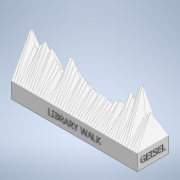
# Autodesk Inventor part: base_fourier
Saved by Autodesk Inventor 2020.1 (Build 241239000, 239)
## iProperties
Created: 2019-10-02
Part Number: base_fourier
Material: Generic
Document SubType Name: Modeling
Designer: Babynado
Density: 1 g/cm^3
Appearance: Default
Author: Babynado
Autodesk Inventor part; units mm, degrees
(part 1 of 3)
ref_plane "YZ Plane" through (0, 0, 0) normal (1, 0, 0) x (0, 1, 0)
ref_plane "XZ Plane" through (0, 0, 0) normal (0, 1, 0) x (-1, 0, 0)
ref_plane "XY Plane" through (0, 0, 0) normal (0, 0, 1) x (1, 0, 0)
sketch "Sketch1" plane through (0, 0, 0) normal (0, 1, 0) x (-1, 0, 0)
  line L0 (0, 50.8) -> (-203.2, 50.8) projected
  line L1 (0, 0) -> (0, 50.8) projected
  line L2 (-203.2, 0) -> (0, 0) projected
  line L3 (-203.2, 50.8) -> (-203.2, 0) projected
extrude "Extrusion1" add sketch "Sketch1" against normal blind 25.4
sketch "Sketch2" plane through (0, 0, 50.8) normal (0, 0, 1) x (1, 0, 0)
  line L0 (0, 0) -> (203.2, 0) projected
  line L1 (0, 0) -> (0, -25.4) projected
  line L2 (203.2, -25.4) -> (0, -25.4) projected
  line L3 (203.2, 0) -> (203.2, -25.4) projected
  line L4 (57.1858, -6.0743) -> (146.0142, -6.0743) construction
  line L5 (146.0142, -6.0743) -> (146.0142, -19.3257) construction
  line L6 (146.0142, -19.3257) -> (57.1858, -19.3257) construction
  line L7 (57.1858, -19.3257) -> (57.1858, -6.0743) construction
  line L8 (65.2204, -17.272) -> (59.9222, -17.272)
  line L9 (59.9222, -17.272) -> (59.9222, -8.128)
  line L10 (59.9222, -8.128) -> (61.1374, -8.128)
  line L11 (61.1374, -8.128) -> (61.1374, -16.1901)
  line L12 (61.1374, -16.1901) -> (65.2204, -16.1901)
  line L13 (65.2204, -16.1901) -> (65.2204, -17.272)
  line L14 (69.3626, -17.272) -> (65.8206, -17.272)
  line L15 (65.8206, -17.272) -> (65.8206, -16.3383)
  line L16 (65.8206, -16.3383) -> (66.984, -16.3383)
  line L17 (66.984, -16.3383) -> (66.984, -9.0617)
  line L18 (66.984, -9.0617) -> (65.8206, -9.0617)
  line L19 (65.8206, -9.0617) -> (65.8206, -8.128)
  line L20 (65.8206, -8.128) -> (69.3626, -8.128)
  line L21 (69.3626, -8.128) -> (69.3626, -9.0617)
  line L22 (69.3626, -9.0617) -> (68.1992, -9.0617)
  line L23 (68.1992, -9.0617) -> (68.1992, -16.3383)
  line L24 (68.1992, -16.3383) -> (69.3626, -16.3383)
  line L25 (69.3626, -16.3383) -> (69.3626, -17.272)
  spline S0 degree 2 poles (77.069, -14.4636) (77.069, -15.1453) (76.5503, -16.1901) (76.1205, -16.531) knots 0 0 0 1 2 2 2
  spline S1 degree 2 poles (76.1205, -16.531) (75.6018, -16.9311) (74.4236, -17.272) (73.49, -17.272) knots 0 0 0 1 2 2 2
  line L26 (73.49, -17.272) -> (70.8668, -17.272)
  line L27 (70.8668, -17.272) -> (70.8668, -8.128)
  line L28 (70.8668, -8.128) -> (73.2899, -8.128)
  spline S2 degree 2 poles (73.2899, -8.128) (74.268, -8.128) (75.2462, -8.254) (75.6908, -8.4985) knots 0 0 0 1 2 2 2
  spline S3 degree 2 poles (75.6908, -8.4985) (76.1872, -8.7579) (76.6392, -9.61) (76.6392, -10.188) knots 0 0 0 1 2 2 2
  spline S4 degree 2 poles (76.6392, -10.188) (76.6392, -10.8327) (75.9575, -11.8553) (75.3573, -12.1442) knots 0 0 0 1 2 2 2
  line L29 (75.3573, -12.1442) -> (75.3573, -12.1887)
  spline S5 degree 2 poles (75.3573, -12.1887) (76.1724, -12.411) (77.069, -13.5892) (77.069, -14.4636) knots 0 0 0 1 2 2 2
  spline S6 degree 2 poles (75.8019, -14.5155) (75.8019, -13.9968) (75.5055, -13.3299) (75.0609, -13.0927) knots 0 0 0 1 2 2 2
  spline S7 degree 2 poles (75.0609, -13.0927) (74.7719, -12.9445) (74.0902, -12.8556) (73.4603, -12.8556) knots 0 0 0 1 2 2 2
  line L30 (73.4603, -12.8556) -> (72.0821, -12.8556)
  line L31 (72.0821, -12.8556) -> (72.0821, -16.2346)
  line L32 (72.0821, -16.2346) -> (73.0676, -16.2346)
  spline S8 degree 2 poles (73.0676, -16.2346) (73.8679, -16.2346) (74.7867, -16.0864) (75.1424, -15.8493) knots 0 0 0 1 2 2 2
  spline S9 degree 2 poles (75.1424, -15.8493) (75.4833, -15.6047) (75.8019, -14.9971) (75.8019, -14.5155) knots 0 0 0 1 2 2 2
  spline S10 degree 2 poles (75.3721, -10.3584) (75.3721, -10.0324) (75.1498, -9.5433) (74.9053, -9.4025) knots 0 0 0 1 2 2 2
  spline S11 degree 2 poles (74.9053, -9.4025) (74.6089, -9.2395) (73.8901, -9.1654) (73.2454, -9.1654) knots 0 0 0 1 2 2 2
  line L33 (73.2454, -9.1654) -> (72.0821, -9.1654)
  line L34 (72.0821, -9.1654) -> (72.0821, -11.8404)
  line L35 (72.0821, -11.8404) -> (73.4603, -11.8404)
  spline S12 degree 2 poles (73.4603, -11.8404) (74.0309, -11.8404) (74.5718, -11.7219) (74.8608, -11.5366) knots 0 0 0 1 2 2 2
  spline S13 degree 2 poles (74.8608, -11.5366) (75.1424, -11.3588) (75.3721, -10.7882) (75.3721, -10.3584) knots 0 0 0 1 2 2 2
  line L36 (85.3535, -17.272) -> (83.7751, -17.272)
  line L37 (83.7751, -17.272) -> (80.8852, -13.6337)
  line L38 (80.8852, -13.6337) -> (79.4921, -13.6337)
  line L39 (79.4921, -13.6337) -> (79.4921, -17.272)
  line L40 (79.4921, -17.272) -> (78.2769, -17.272)
  line L41 (78.2769, -17.272) -> (78.2769, -8.128)
  line L42 (78.2769, -8.128) -> (80.6333, -8.128)
  spline S14 degree 2 poles (80.6333, -8.128) (81.4187, -8.128) (82.4784, -8.2984) (82.96, -8.6097) knots 0 0 0 1 2 2 2
  spline S15 degree 2 poles (82.96, -8.6097) (83.4417, -8.9209) (83.9974, -9.8916) (83.9974, -10.6104) knots 0 0 0 1 2 2 2
  spline S16 degree 2 poles (83.9974, -10.6104) (83.9974, -11.6107) (82.9748, -12.9668) (82.1005, -13.2928) knots 0 0 0 1 2 2 2
  line L43 (82.1005, -13.2928) -> (85.3535, -17.272)
  spline S17 degree 2 poles (82.7303, -10.7067) (82.7303, -10.3066) (82.4487, -9.6915) (82.1523, -9.4914) knots 0 0 0 1 2 2 2
  spline S18 degree 2 poles (82.1523, -9.4914) (81.893, -9.321) (81.2038, -9.1802) (80.7, -9.1802) knots 0 0 0 1 2 2 2
  line L44 (80.7, -9.1802) -> (79.4921, -9.1802)
  line L45 (79.4921, -9.1802) -> (79.4921, -12.6185)
  line L46 (79.4921, -12.6185) -> (80.5592, -12.6185)
  spline S19 degree 2 poles (80.5592, -12.6185) (81.0853, -12.6185) (81.9226, -12.4332) (82.2116, -12.1442) knots 0 0 0 1 2 2 2
  spline S20 degree 2 poles (82.2116, -12.1442) (82.4784, -11.8923) (82.7303, -11.1809) (82.7303, -10.7067) knots 0 0 0 1 2 2 2
  line L47 (85.0941, -17.272) -> (88.1767, -8.128)
  line L48 (88.1767, -8.128) -> (89.6735, -8.128)
  line L49 (89.6735, -8.128) -> (92.7561, -17.272)
  line L50 (92.7561, -17.272) -> (91.4742, -17.272)
  line L51 (91.4742, -17.272) -> (90.6442, -14.7155)
  line L52 (90.6442, -14.7155) -> (87.1541, -14.7155)
  line L53 (87.1541, -14.7155) -> (86.3242, -17.272)
  line L54 (86.3242, -17.272) -> (85.0941, -17.272)
  line L55 (90.3108, -13.6781) -> (88.8955, -9.3729)
  line L56 (88.8955, -9.3729) -> (87.4876, -13.6781)
  line L57 (87.4876, -13.6781) -> (90.3108, -13.6781)
  line L58 (100.6997, -17.272) -> (99.1213, -17.272)
  line L59 (99.1213, -17.272) -> (96.2314, -13.6337)
  line L60 (96.2314, -13.6337) -> (94.8383, -13.6337)
  line L61 (94.8383, -13.6337) -> (94.8383, -17.272)
  line L62 (94.8383, -17.272) -> (93.6231, -17.272)
  line L63 (93.6231, -17.272) -> (93.6231, -8.128)
  line L64 (93.6231, -8.128) -> (95.9795, -8.128)
  spline S21 degree 2 poles (95.9795, -8.128) (96.7649, -8.128) (97.8246, -8.2984) (98.3062, -8.6097) knots 0 0 0 1 2 2 2
  spline S22 degree 2 poles (98.3062, -8.6097) (98.7879, -8.9209) (99.3436, -9.8916) (99.3436, -10.6104) knots 0 0 0 1 2 2 2
  spline S23 degree 2 poles (99.3436, -10.6104) (99.3436, -11.6107) (98.3211, -12.9668) (97.4467, -13.2928) knots 0 0 0 1 2 2 2
  line L65 (97.4467, -13.2928) -> (100.6997, -17.272)
  spline S24 degree 2 poles (98.0765, -10.7067) (98.0765, -10.3066) (97.7949, -9.6915) (97.4985, -9.4914) knots 0 0 0 1 2 2 2
  spline S25 degree 2 poles (97.4985, -9.4914) (97.2392, -9.321) (96.55, -9.1802) (96.0462, -9.1802) knots 0 0 0 1 2 2 2
  line L66 (96.0462, -9.1802) -> (94.8383, -9.1802)
  line L67 (94.8383, -9.1802) -> (94.8383, -12.6185)
  line L68 (94.8383, -12.6185) -> (95.9054, -12.6185)
  spline S26 degree 2 poles (95.9054, -12.6185) (96.4315, -12.6185) (97.2688, -12.4332) (97.5578, -12.1442) knots 0 0 0 1 2 2 2
  spline S27 degree 2 poles (97.5578, -12.1442) (97.8246, -11.8923) (98.0765, -11.1809) (98.0765, -10.7067) knots 0 0 0 1 2 2 2
  line L69 (107.8281, -8.128) -> (104.7382, -13.2261)
  line L70 (104.7382, -13.2261) -> (104.7382, -17.272)
  line L71 (104.7382, -17.272) -> (103.5229, -17.272)
  line L72 (103.5229, -17.272) -> (103.5229, -13.3521)
  line L73 (103.5229, -13.3521) -> (100.4329, -8.128)
  line L74 (100.4329, -8.128) -> (101.7815, -8.128)
  line L75 (101.7815, -8.128) -> (104.1379, -12.1517)
  line L76 (104.1379, -12.1517) -> (106.5388, -8.128)
  line L77 (106.5388, -8.128) -> (107.8281, -8.128)
  line L78 (122.8483, -8.128) -> (120.5512, -17.272)
  line L79 (120.5512, -17.272) -> (119.1877, -17.272)
  line L80 (119.1877, -17.272) -> (117.3278, -9.6841)
  line L81 (117.3278, -9.6841) -> (115.5198, -17.272)
  line L82 (115.5198, -17.272) -> (114.1711, -17.272)
  line L83 (114.1711, -17.272) -> (111.837, -8.128)
  line L84 (111.837, -8.128) -> (113.0893, -8.128)
  line L85 (113.0893, -8.128) -> (114.927, -15.7085)
  line L86 (114.927, -15.7085) -> (116.7498, -8.128)
  line L87 (116.7498, -8.128) -> (117.9873, -8.128)
  line L88 (117.9873, -8.128) -> (119.825, -15.7974)
  line L89 (119.825, -15.7974) -> (121.6553, -8.128)
  line L90 (121.6553, -8.128) -> (122.8483, -8.128)
  line L91 (122.9521, -17.272) -> (126.0346, -8.128)
  line L92 (126.0346, -8.128) -> (127.5315, -8.128)
  line L93 (127.5315, -8.128) -> (130.614, -17.272)
  line L94 (130.614, -17.272) -> (129.3321, -17.272)
  line L95 (129.3321, -17.272) -> (128.5022, -14.7155)
  line L96 (128.5022, -14.7155) -> (125.012, -14.7155)
  line L97 (125.012, -14.7155) -> (124.1821, -17.272)
  line L98 (124.1821, -17.272) -> (122.9521, -17.272)
  line L99 (128.1687, -13.6781) -> (126.7534, -9.3729)
  line L100 (126.7534, -9.3729) -> (125.3455, -13.6781)
  line L101 (125.3455, -13.6781) -> (128.1687, -13.6781)
  line L102 (136.7792, -17.272) -> (131.481, -17.272)
  line L103 (131.481, -17.272) -> (131.481, -8.128)
  line L104 (131.481, -8.128) -> (132.6963, -8.128)
  line L105 (132.6963, -8.128) -> (132.6963, -16.1901)
  line L106 (132.6963, -16.1901) -> (136.7792, -16.1901)
  line L107 (136.7792, -16.1901) -> (136.7792, -17.272)
  line L108 (144.4041, -17.272) -> (142.8258, -17.272)
  line L109 (142.8258, -17.272) -> (139.4839, -13.0186)
  line L110 (139.4839, -13.0186) -> (138.9503, -13.6188)
  line L111 (138.9503, -13.6188) -> (138.9503, -17.272)
  line L112 (138.9503, -17.272) -> (137.7351, -17.272)
  line L113 (137.7351, -17.272) -> (137.7351, -8.128)
  line L114 (137.7351, -8.128) -> (138.9503, -8.128)
  line L115 (138.9503, -8.128) -> (138.9503, -12.3295)
  line L116 (138.9503, -12.3295) -> (142.6998, -8.128)
  line L117 (142.6998, -8.128) -> (144.1818, -8.128)
  line L118 (144.1818, -8.128) -> (140.3953, -12.2109)
  line L119 (140.3953, -12.2109) -> (144.4041, -17.272)
  dimension "d2" = 203.2
  dimension "d3" = 25.4
  dimension "d4" = 88.8284
  dimension "d5" = 13.2514
  dimension "d6" = 6.0743
  dimension "d7" = 57.1858
  constraints: 2 other
  measures "d2" distance of L0.start L0.end
  measures "d3" distance of L0.start L1.end
  measures "d4" distance of L4.start L4.end
  measures "d5" distance of L6.end L4.start
  measures "d6" distance between parallel lines of L0 L4
  measures "d7" distance between parallel lines of L1 L7
extrude "Extrusion2" cut sketch "Sketch2" against normal blind 5.08 contours L8 L9 L10 L11 L12 L13 | L14 L15 L16 L17 L18 L19 L20 L21 L22 L23 L24 L25 | S0 S1 L26 L27 L28 S2 S3 S4 L29 S5 | L36 L47 L43 | L43 L47 L48 L49 L50 L51 L52 L53 L54 | L36 L37 L38 L39 L40 L41 L42 S14 S15 S16 L43 L47 | L58 L59 L60 L61 L62 L63 L64 S21 S22 S23 L65 | L69 L70 L71 L72 L73 L74 L75 L76 L77 | L78 L79 L80 L81 L82 L83 L84 L85 L86 L87 L88 L89 L90 | L91 L92 L93 L94 L95 L96 L97 L98 | L102 L103 L104 L105 L106 L107 | L108 L109 L110 L111 L112 L113 L114 L115 L116 L117 L118 L119
sketch "Sketch3" plane through (0, -25.4, 0) normal (0, -1, 0) x (1, 0, 0)
  line L0 (203.2, 0) -> (203.2, 50.8) projected
  line L1 (203.2, 50.8) -> (0, 50.8) projected
  line L2 (0, 50.8) -> (0, 0) projected
  line L3 (0, 0) -> (203.2, 0) projected
  line L4 (6.672, 48.1679) -> (109.1926, 48.1679) construction
  line L5 (109.1926, 48.1679) -> (109.1926, 2.6321) construction
  line L6 (109.1926, 2.6321) -> (6.672, 2.6321) construction
  line L7 (6.672, 2.6321) -> (6.672, 48.1679) construction
  line L8 (115.8646, 37.7597) -> (196.528, 37.7597) construction
  line L9 (196.528, 37.7597) -> (196.528, 13.0403) construction
  line L10 (196.528, 13.0403) -> (115.8646, 13.0403) construction
  line L11 (115.8646, 13.0403) -> (115.8646, 37.7597) construction
  spline S0 degree 2 poles (22.1307, 39.4772) (22.1307, 38.2768) (20.6635, 36.9726) (19.426, 36.9726) knots 0 0 0 1 2 2 2
  spline S1 degree 2 poles (19.426, 36.9726) (19.1296, 36.9726) (18.144, 37.0764) (17.8106, 37.1505) knots 0 0 0 1 2 2 2
  line L12 (17.8106, 37.1505) -> (17.8106, 38.3213)
  line L13 (17.8106, 38.3213) -> (17.8773, 38.3213)
  spline S2 degree 2 poles (17.8773, 38.3213) (18.1292, 38.2323) (18.8776, 38.0249) (19.263, 38.0249) knots 0 0 0 1 2 2 2
  spline S3 degree 2 poles (19.263, 38.0249) (19.8261, 38.0249) (20.5004, 38.2842) (20.6561, 38.5213) knots 0 0 0 1 2 2 2
  spline S4 degree 2 poles (20.6561, 38.5213) (20.8265, 38.7659) (20.9154, 39.4772) (20.9154, 39.9441) knots 0 0 0 1 2 2 2
  line L14 (20.9154, 39.9441) -> (20.9154, 45.2719)
  line L15 (20.9154, 45.2719) -> (18.9814, 45.2719)
  line L16 (18.9814, 45.2719) -> (18.9814, 46.2426)
  line L17 (18.9814, 46.2426) -> (22.1307, 46.2426)
  line L18 (22.1307, 46.2426) -> (22.1307, 39.4772)
  spline S5 degree 2 poles (27.1176, 36.9059) (26.3099, 36.9059) (25.1095, 37.3283) (24.6871, 37.7507) knots 0 0 0 1 2 2 2
  spline S6 degree 2 poles (24.6871, 37.7507) (24.2055, 38.2249) (23.8127, 39.5587) (23.8127, 40.5369) knots 0 0 0 1 2 2 2
  line L19 (23.8127, 40.5369) -> (23.8127, 46.2426)
  line L20 (23.8127, 46.2426) -> (25.028, 46.2426)
  line L21 (25.028, 46.2426) -> (25.028, 40.5369)
  spline S7 degree 2 poles (25.028, 40.5369) (25.028, 39.8996) (25.191, 39.04) (25.4207, 38.6918) knots 0 0 0 1 2 2 2
  spline S8 degree 2 poles (25.4207, 38.6918) (25.6652, 38.3213) (26.51, 37.9433) (27.1176, 37.9433) knots 0 0 0 1 2 2 2
  spline S9 degree 2 poles (27.1176, 37.9433) (27.6882, 37.9433) (28.5774, 38.3213) (28.8219, 38.6918) knots 0 0 0 1 2 2 2
  spline S10 degree 2 poles (28.8219, 38.6918) (29.0516, 39.04) (29.2147, 39.8922) (29.2147, 40.5072) knots 0 0 0 1 2 2 2
  line L22 (29.2147, 40.5072) -> (29.2147, 46.2426)
  line L23 (29.2147, 46.2426) -> (30.4299, 46.2426)
  line L24 (30.4299, 46.2426) -> (30.4299, 40.5369)
  spline S11 degree 2 poles (30.4299, 40.5369) (30.4299, 39.581) (30.0446, 38.2175) (29.5555, 37.7507) knots 0 0 0 1 2 2 2
  spline S12 degree 2 poles (29.5555, 37.7507) (29.1183, 37.3209) (27.9624, 36.9059) (27.1176, 36.9059) knots 0 0 0 1 2 2 2
  spline S13 degree 2 poles (34.7203, 36.9356) (33.7274, 36.9356) (32.3343, 37.3505) (31.7193, 37.6469) knots 0 0 0 1 2 2 2
  line L25 (31.7193, 37.6469) -> (31.7193, 39.1734)
  line L26 (31.7193, 39.1734) -> (31.8082, 39.1734)
  spline S14 degree 2 poles (31.8082, 39.1734) (32.4084, 38.6103) (33.9274, 37.9878) (34.6314, 37.9878) knots 0 0 0 1 2 2 2
  spline S15 degree 2 poles (34.6314, 37.9878) (35.6392, 37.9878) (36.6692, 38.8251) (36.6692, 39.5143) knots 0 0 0 1 2 2 2
  spline S16 degree 2 poles (36.6692, 39.5143) (36.6692, 40.0626) (36.1282, 40.7443) (35.5428, 40.9148) knots 0 0 0 1 2 2 2
  spline S17 degree 2 poles (35.5428, 40.9148) (35.1205, 41.0333) (34.4165, 41.1964) (33.8904, 41.3297) knots 0 0 0 1 2 2 2
  spline S18 degree 2 poles (33.8904, 41.3297) (33.4162, 41.4557) (32.6677, 41.8336) (32.3787, 42.1374) knots 0 0 0 1 2 2 2
  spline S19 degree 2 poles (32.3787, 42.1374) (32.0972, 42.4412) (31.7859, 43.2564) (31.7859, 43.7899) knots 0 0 0 1 2 2 2
  spline S20 degree 2 poles (31.7859, 43.7899) (31.7859, 44.9014) (33.5199, 46.4056) (34.8611, 46.4056) knots 0 0 0 1 2 2 2
  spline S21 degree 2 poles (34.8611, 46.4056) (35.6318, 46.4056) (36.9952, 46.1018) (37.5806, 45.8128) knots 0 0 0 1 2 2 2
  line L27 (37.5806, 45.8128) -> (37.5806, 44.3605)
  line L28 (37.5806, 44.3605) -> (37.4917, 44.3605)
  spline S22 degree 2 poles (37.4917, 44.3605) (37.0545, 44.7606) (35.691, 45.3534) (34.9426, 45.3534) knots 0 0 0 1 2 2 2
  spline S23 degree 2 poles (34.9426, 45.3534) (34.0979, 45.3534) (33.0531, 44.5605) (33.0531, 43.9158) knots 0 0 0 1 2 2 2
  spline S24 degree 2 poles (33.0531, 43.9158) (33.0531, 43.3379) (33.6681, 42.6487) (34.2461, 42.4931) knots 0 0 0 1 2 2 2
  spline S25 degree 2 poles (34.2461, 42.4931) (34.6314, 42.3894) (35.7503, 42.1226) (36.1208, 42.0115) knots 0 0 0 1 2 2 2
  spline S26 degree 2 poles (36.1208, 42.0115) (37.0619, 41.7225) (37.9363, 40.5591) (37.9363, 39.7069) knots 0 0 0 1 2 2 2
  spline S27 degree 2 poles (37.9363, 39.7069) (37.9363, 39.166) (37.4991, 38.1286) (37.1064, 37.7655) knots 0 0 0 1 2 2 2
  spline S28 degree 2 poles (37.1064, 37.7655) (36.6692, 37.3654) (35.5577, 36.9356) (34.7203, 36.9356) knots 0 0 0 1 2 2 2
  line L29 (41.3079, 37.0986) -> (41.3079, 45.1607)
  line L30 (41.3079, 45.1607) -> (38.2401, 45.1607)
  line L31 (38.2401, 45.1607) -> (38.2401, 46.2426)
  line L32 (38.2401, 46.2426) -> (45.5909, 46.2426)
  line L33 (45.5909, 46.2426) -> (45.5909, 45.1607)
  line L34 (45.5909, 45.1607) -> (42.5231, 45.1607)
  line L35 (42.5231, 45.1607) -> (42.5231, 37.0986)
  line L36 (42.5231, 37.0986) -> (41.3079, 37.0986)
  line L37 (49.7034, 37.0986) -> (46.1614, 37.0986)
  line L38 (46.1614, 37.0986) -> (46.1614, 38.0323)
  line L39 (46.1614, 38.0323) -> (47.3248, 38.0323)
  line L40 (47.3248, 38.0323) -> (47.3248, 45.3089)
  line L41 (47.3248, 45.3089) -> (46.1614, 45.3089)
  line L42 (46.1614, 45.3089) -> (46.1614, 46.2426)
  line L43 (46.1614, 46.2426) -> (49.7034, 46.2426)
  line L44 (49.7034, 46.2426) -> (49.7034, 45.3089)
  line L45 (49.7034, 45.3089) -> (48.5401, 45.3089)
  line L46 (48.5401, 45.3089) -> (48.5401, 38.0323)
  line L47 (48.5401, 38.0323) -> (49.7034, 38.0323)
  line L48 (49.7034, 38.0323) -> (49.7034, 37.0986)
  line L49 (57.7508, 37.0986) -> (56.3873, 37.0986)
  line L50 (56.3873, 37.0986) -> (52.3414, 44.9829)
  line L51 (52.3414, 44.9829) -> (52.3414, 37.0986)
  line L52 (52.3414, 37.0986) -> (51.2077, 37.0986)
  line L53 (51.2077, 37.0986) -> (51.2077, 46.2426)
  line L54 (51.2077, 46.2426) -> (52.9342, 46.2426)
  line L55 (52.9342, 46.2426) -> (56.617, 39.003)
  line L56 (56.617, 39.003) -> (56.617, 46.2426)
  line L57 (56.617, 46.2426) -> (57.7508, 46.2426)
  line L58 (57.7508, 46.2426) -> (57.7508, 37.0986)
  line L59 (62.5451, 37.0986) -> (65.6276, 46.2426)
  line L60 (65.6276, 46.2426) -> (67.1245, 46.2426)
  line L61 (67.1245, 46.2426) -> (70.207, 37.0986)
  line L62 (70.207, 37.0986) -> (68.9251, 37.0986)
  line L63 (68.9251, 37.0986) -> (68.0952, 39.6551)
  line L64 (68.0952, 39.6551) -> (64.605, 39.6551)
  line L65 (64.605, 39.6551) -> (63.7751, 37.0986)
  line L66 (63.7751, 37.0986) -> (62.5451, 37.0986)
  line L67 (67.7617, 40.6925) -> (66.3464, 44.9977)
  line L68 (66.3464, 44.9977) -> (64.9385, 40.6925)
  line L69 (64.9385, 40.6925) -> (67.7617, 40.6925)
  line L70 (76.3722, 37.0986) -> (71.074, 37.0986)
  line L71 (71.074, 37.0986) -> (71.074, 46.2426)
  line L72 (71.074, 46.2426) -> (72.2893, 46.2426)
  line L73 (72.2893, 46.2426) -> (72.2893, 38.1805)
  line L74 (72.2893, 38.1805) -> (76.3722, 38.1805)
  line L75 (76.3722, 38.1805) -> (76.3722, 37.0986)
  line L76 (82.6263, 37.0986) -> (77.3281, 37.0986)
  line L77 (77.3281, 37.0986) -> (77.3281, 46.2426)
  line L78 (77.3281, 46.2426) -> (78.5433, 46.2426)
  line L79 (78.5433, 46.2426) -> (78.5433, 38.1805)
  line L80 (78.5433, 38.1805) -> (82.6263, 38.1805)
  line L81 (82.6263, 38.1805) -> (82.6263, 37.0986)
  line L82 (83.5822, 37.0986) -> (83.5822, 46.2426)
  line L83 (83.5822, 46.2426) -> (89.3027, 46.2426)
  line L84 (89.3027, 46.2426) -> (89.3027, 45.1607)
  line L85 (89.3027, 45.1607) -> (84.7974, 45.1607)
  line L86 (84.7974, 45.1607) -> (84.7974, 42.6561)
  line L87 (84.7974, 42.6561) -> (88.9989, 42.6561)
  line L88 (88.9989, 42.6561) -> (88.9989, 41.5743)
  line L89 (88.9989, 41.5743) -> (84.7974, 41.5743)
  line L90 (84.7974, 41.5743) -> (84.7974, 38.1805)
  line L91 (84.7974, 38.1805) -> (89.3027, 38.1805)
  line L92 (89.3027, 38.1805) -> (89.3027, 37.0986)
  line L93 (89.3027, 37.0986) -> (83.5822, 37.0986)
  line L94 (97.1796, 37.0986) -> (95.8162, 37.0986)
  line L95 (95.8162, 37.0986) -> (91.7703, 44.9829)
  line L96 (91.7703, 44.9829) -> (91.7703, 37.0986)
  line L97 (91.7703, 37.0986) -> (90.6365, 37.0986)
  line L98 (90.6365, 37.0986) -> (90.6365, 46.2426)
  line L99 (90.6365, 46.2426) -> (92.3631, 46.2426)
  line L100 (92.3631, 46.2426) -> (96.0459, 39.003)
  line L101 (96.0459, 39.003) -> (96.0459, 46.2426)
  line L102 (96.0459, 46.2426) -> (97.1796, 46.2426)
  line L103 (97.1796, 46.2426) -> (97.1796, 37.0986)
  line L104 (26.6545, 22.0432) -> (29.7371, 31.1872)
  line L105 (29.7371, 31.1872) -> (31.2339, 31.1872)
  line L106 (31.2339, 31.1872) -> (34.3165, 22.0432)
  line L107 (34.3165, 22.0432) -> (33.0345, 22.0432)
  line L108 (33.0345, 22.0432) -> (32.2046, 24.5997)
  line L109 (32.2046, 24.5997) -> (28.7145, 24.5997)
  line L110 (28.7145, 24.5997) -> (27.8846, 22.0432)
  line L111 (27.8846, 22.0432) -> (26.6545, 22.0432)
  line L112 (31.8712, 25.6371) -> (30.4558, 29.9424)
  line L113 (30.4558, 29.9424) -> (29.0479, 25.6371)
  line L114 (29.0479, 25.6371) -> (31.8712, 25.6371)
  line L115 (40.1037, 22.0432) -> (35.6429, 22.0432)
  line L116 (35.6429, 22.0432) -> (35.6429, 22.9769)
  line L117 (35.6429, 22.9769) -> (37.3027, 22.9769)
  line L118 (37.3027, 22.9769) -> (37.3027, 29.105)
  line L119 (37.3027, 29.105) -> (35.6429, 29.105)
  line L120 (35.6429, 29.105) -> (35.6429, 29.9424)
  spline S29 degree 2 poles (35.6429, 29.9424) (36.584, 29.9424) (37.4732, 30.4759) (37.5324, 31.2169) knots 0 0 0 1 2 2 2
  line L121 (37.5324, 31.2169) -> (38.4809, 31.2169)
  line L122 (38.4809, 31.2169) -> (38.4809, 22.9769)
  line L123 (38.4809, 22.9769) -> (40.1037, 22.9769)
  line L124 (40.1037, 22.9769) -> (40.1037, 22.0432)
  line L125 (47.6694, 25.1851) -> (46.5801, 25.1851)
  line L126 (46.5801, 25.1851) -> (46.5801, 22.0432)
  line L127 (46.5801, 22.0432) -> (45.4019, 22.0432)
  line L128 (45.4019, 22.0432) -> (45.4019, 25.1851)
  line L129 (45.4019, 25.1851) -> (41.3634, 25.1851)
  line L130 (41.3634, 25.1851) -> (41.3634, 26.4745)
  line L131 (41.3634, 26.4745) -> (45.4538, 31.1872)
  line L132 (45.4538, 31.1872) -> (46.5801, 31.1872)
  line L133 (46.5801, 31.1872) -> (46.5801, 26.1706)
  line L134 (46.5801, 26.1706) -> (47.6694, 26.1706)
  line L135 (47.6694, 26.1706) -> (47.6694, 25.1851)
  line L136 (45.4019, 26.1706) -> (45.4019, 29.7423)
  line L137 (45.4019, 29.7423) -> (42.3267, 26.1706)
  line L138 (42.3267, 26.1706) -> (45.4019, 26.1706)
  spline S30 degree 2 poles (54.1902, 24.948) (54.1902, 24.2885) (53.7679, 23.1622) (53.3825, 22.7472) knots 0 0 0 1 2 2 2
  spline S31 degree 2 poles (53.3825, 22.7472) (52.9972, 22.3322) (51.8487, 21.8506) (51.1373, 21.8506) knots 0 0 0 1 2 2 2
  spline S32 degree 2 poles (51.1373, 21.8506) (50.4852, 21.8506) (49.2107, 22.1396) (48.7438, 22.3693) knots 0 0 0 1 2 2 2
  line L139 (48.7438, 22.3693) -> (48.7438, 23.666)
  line L140 (48.7438, 23.666) -> (48.8328, 23.666)
  spline S33 degree 2 poles (48.8328, 23.666) (48.9736, 23.5623) (49.4997, 23.2955) (49.8183, 23.177) knots 0 0 0 1 2 2 2
  spline S34 degree 2 poles (49.8183, 23.177) (50.1814, 23.051) (50.7816, 22.9102) (51.1595, 22.9102) knots 0 0 0 1 2 2 2
  spline S35 degree 2 poles (51.1595, 22.9102) (51.53, 22.9102) (52.2266, 23.177) (52.4785, 23.466) knots 0 0 0 1 2 2 2
  spline S36 degree 2 poles (52.4785, 23.466) (52.7082, 23.7401) (52.9453, 24.4663) (52.9453, 24.9554) knots 0 0 0 1 2 2 2
  spline S37 degree 2 poles (52.9453, 24.9554) (52.9453, 25.4445) (52.6786, 26.0669) (52.4266, 26.2744) knots 0 0 0 1 2 2 2
  spline S38 degree 2 poles (52.4266, 26.2744) (52.1673, 26.5041) (51.3966, 26.6968) (50.9298, 26.6968) knots 0 0 0 1 2 2 2
  spline S39 degree 2 poles (50.9298, 26.6968) (50.4259, 26.6968) (49.4256, 26.5411) (49.1218, 26.4745) knots 0 0 0 1 2 2 2
  line L141 (49.1218, 26.4745) -> (49.1218, 31.1872)
  line L142 (49.1218, 31.1872) -> (54.1384, 31.1872)
  line L143 (54.1384, 31.1872) -> (54.1384, 30.1128)
  line L144 (54.1384, 30.1128) -> (50.3, 30.1128)
  line L145 (50.3, 30.1128) -> (50.3, 27.6749)
  spline S40 degree 2 poles (50.3, 27.6749) (50.5223, 27.7045) (50.952, 27.7268) (51.1299, 27.7268) knots 0 0 0 1 2 2 2
  spline S41 degree 2 poles (51.1299, 27.7268) (51.8338, 27.7268) (52.8045, 27.497) (53.2492, 27.1562) knots 0 0 0 1 2 2 2
  spline S42 degree 2 poles (53.2492, 27.1562) (53.7012, 26.8153) (54.1902, 25.7779) (54.1902, 24.948) knots 0 0 0 1 2 2 2
  spline S43 degree 2 poles (61.2891, 25.0073) (61.2891, 24.3033) (60.8222, 23.1103) (60.4295, 22.7102) knots 0 0 0 1 2 2 2
  spline S44 degree 2 poles (60.4295, 22.7102) (60.0219, 22.2878) (58.9993, 21.8506) (58.3843, 21.8506) knots 0 0 0 1 2 2 2
  spline S45 degree 2 poles (58.3843, 21.8506) (57.7693, 21.8506) (56.7541, 22.2655) (56.3688, 22.6805) knots 0 0 0 1 2 2 2
  spline S46 degree 2 poles (56.3688, 22.6805) (55.8945, 23.177) (55.361, 24.8442) (55.361, 26.0595) knots 0 0 0 1 2 2 2
  spline S47 degree 2 poles (55.361, 26.0595) (55.361, 27.2525) (55.8501, 29.1717) (56.3614, 29.8831) knots 0 0 0 1 2 2 2
  spline S48 degree 2 poles (56.3614, 29.8831) (56.8578, 30.5796) (58.4288, 31.3577) (59.4588, 31.3577) knots 0 0 0 1 2 2 2
  spline S49 degree 2 poles (59.4588, 31.3577) (59.7626, 31.3577) (60.2961, 31.2984) (60.4962, 31.2317) knots 0 0 0 1 2 2 2
  line L146 (60.4962, 31.2317) -> (60.4962, 30.0535)
  line L147 (60.4962, 30.0535) -> (60.4443, 30.0535)
  spline S50 degree 2 poles (60.4443, 30.0535) (60.2739, 30.1424) (59.6514, 30.298) (59.2957, 30.298) knots 0 0 0 1 2 2 2
  spline S51 degree 2 poles (59.2957, 30.298) (58.1546, 30.298) (56.7541, 28.7568) (56.6207, 27.2451) knots 0 0 0 1 2 2 2
  spline S52 degree 2 poles (56.6207, 27.2451) (57.0579, 27.5489) (57.9768, 27.8824) (58.5251, 27.8824) knots 0 0 0 1 2 2 2
  spline S53 degree 2 poles (58.5251, 27.8824) (59.0586, 27.8824) (59.8589, 27.6675) (60.2961, 27.3414) knots 0 0 0 1 2 2 2
  spline S54 degree 2 poles (60.2961, 27.3414) (60.8, 26.9635) (61.2891, 25.7927) (61.2891, 25.0073) knots 0 0 0 1 2 2 2
  spline S55 degree 2 poles (60.0442, 24.9554) (60.0442, 25.5186) (59.7478, 26.2818) (59.4217, 26.5486) knots 0 0 0 1 2 2 2
  spline S56 degree 2 poles (59.4217, 26.5486) (59.1772, 26.7412) (58.5696, 26.8672) (58.2509, 26.8672) knots 0 0 0 1 2 2 2
  spline S57 degree 2 poles (58.2509, 26.8672) (57.8212, 26.8672) (57.0135, 26.6078) (56.6207, 26.3633) knots 0 0 0 1 2 2 2
  spline S58 degree 2 poles (56.6207, 26.3633) (56.6133, 26.2299) (56.5985, 25.978) (56.5985, 25.7853) knots 0 0 0 1 2 2 2
  spline S59 degree 2 poles (56.5985, 25.7853) (56.5985, 24.8368) (56.969, 23.6735) (57.2506, 23.3696) knots 0 0 0 1 2 2 2
  spline S60 degree 2 poles (57.2506, 23.3696) (57.5099, 23.0807) (58.0731, 22.8509) (58.3917, 22.8509) knots 0 0 0 1 2 2 2
  spline S61 degree 2 poles (58.3917, 22.8509) (59.1327, 22.8509) (60.0442, 23.9032) (60.0442, 24.9554) knots 0 0 0 1 2 2 2
  spline S62 degree 2 poles (68.1508, 25.0073) (68.1508, 24.3033) (67.6839, 23.1103) (67.2912, 22.7102) knots 0 0 0 1 2 2 2
  spline S63 degree 2 poles (67.2912, 22.7102) (66.8836, 22.2878) (65.8611, 21.8506) (65.246, 21.8506) knots 0 0 0 1 2 2 2
  spline S64 degree 2 poles (65.246, 21.8506) (64.631, 21.8506) (63.6158, 22.2655) (63.2305, 22.6805) knots 0 0 0 1 2 2 2
  spline S65 degree 2 poles (63.2305, 22.6805) (62.7562, 23.177) (62.2227, 24.8442) (62.2227, 26.0595) knots 0 0 0 1 2 2 2
  spline S66 degree 2 poles (62.2227, 26.0595) (62.2227, 27.2525) (62.7118, 29.1717) (63.2231, 29.8831) knots 0 0 0 1 2 2 2
  spline S67 degree 2 poles (63.2231, 29.8831) (63.7195, 30.5796) (65.2905, 31.3577) (66.3205, 31.3577) knots 0 0 0 1 2 2 2
  spline S68 degree 2 poles (66.3205, 31.3577) (66.6243, 31.3577) (67.1578, 31.2984) (67.3579, 31.2317) knots 0 0 0 1 2 2 2
  line L148 (67.3579, 31.2317) -> (67.3579, 30.0535)
  line L149 (67.3579, 30.0535) -> (67.306, 30.0535)
  spline S69 degree 2 poles (67.306, 30.0535) (67.1356, 30.1424) (66.5131, 30.298) (66.1575, 30.298) knots 0 0 0 1 2 2 2
  spline S70 degree 2 poles (66.1575, 30.298) (65.0163, 30.298) (63.6158, 28.7568) (63.4824, 27.2451) knots 0 0 0 1 2 2 2
  spline S71 degree 2 poles (63.4824, 27.2451) (63.9196, 27.5489) (64.8385, 27.8824) (65.3868, 27.8824) knots 0 0 0 1 2 2 2
  spline S72 degree 2 poles (65.3868, 27.8824) (65.9203, 27.8824) (66.7206, 27.6675) (67.1578, 27.3414) knots 0 0 0 1 2 2 2
  spline S73 degree 2 poles (67.1578, 27.3414) (67.6617, 26.9635) (68.1508, 25.7927) (68.1508, 25.0073) knots 0 0 0 1 2 2 2
  spline S74 degree 2 poles (66.9059, 24.9554) (66.9059, 25.5186) (66.6095, 26.2818) (66.2834, 26.5486) knots 0 0 0 1 2 2 2
  spline S75 degree 2 poles (66.2834, 26.5486) (66.0389, 26.7412) (65.4313, 26.8672) (65.1126, 26.8672) knots 0 0 0 1 2 2 2
  spline S76 degree 2 poles (65.1126, 26.8672) (64.6829, 26.8672) (63.8752, 26.6078) (63.4824, 26.3633) knots 0 0 0 1 2 2 2
  spline S77 degree 2 poles (63.4824, 26.3633) (63.475, 26.2299) (63.4602, 25.978) (63.4602, 25.7853) knots 0 0 0 1 2 2 2
  spline S78 degree 2 poles (63.4602, 25.7853) (63.4602, 24.8368) (63.8307, 23.6735) (64.1123, 23.3696) knots 0 0 0 1 2 2 2
  spline S79 degree 2 poles (64.1123, 23.3696) (64.3716, 23.0807) (64.9348, 22.8509) (65.2534, 22.8509) knots 0 0 0 1 2 2 2
  spline S80 degree 2 poles (65.2534, 22.8509) (65.9944, 22.8509) (66.9059, 23.9032) (66.9059, 24.9554) knots 0 0 0 1 2 2 2
  spline S81 degree 2 poles (74.9235, 26.6152) (74.9235, 24.1551) (73.4934, 21.8506) (72.004, 21.8506) knots 0 0 0 1 2 2 2
  spline S82 degree 2 poles (72.004, 21.8506) (70.4923, 21.8506) (69.077, 24.1996) (69.077, 26.6078) knots 0 0 0 1 2 2 2
  spline S83 degree 2 poles (69.077, 26.6078) (69.077, 29.0828) (70.5072, 31.3725) (72.004, 31.3725) knots 0 0 0 1 2 2 2
  spline S84 degree 2 poles (72.004, 31.3725) (73.5082, 31.3725) (74.9235, 29.0013) (74.9235, 26.6152) knots 0 0 0 1 2 2 2
  spline S85 degree 2 poles (73.3526, 23.8291) (73.5305, 24.2811) (73.6787, 25.6742) (73.6787, 26.6152) knots 0 0 0 1 2 2 2
  spline S86 degree 2 poles (73.6787, 26.6152) (73.6787, 27.5563) (73.5305, 28.942) (73.3452, 29.4088) knots 0 0 0 1 2 2 2
  spline S87 degree 2 poles (73.3452, 29.4088) (73.16, 29.8757) (72.5153, 30.3573) (72.004, 30.3573) knots 0 0 0 1 2 2 2
  spline S88 degree 2 poles (72.004, 30.3573) (71.4927, 30.3573) (70.8332, 29.8757) (70.6405, 29.394) knots 0 0 0 1 2 2 2
  spline S89 degree 2 poles (70.6405, 29.394) (70.4553, 28.9272) (70.3219, 27.5045) (70.3219, 26.6078) knots 0 0 0 1 2 2 2
  spline S90 degree 2 poles (70.3219, 26.6078) (70.3219, 25.6445) (70.4405, 24.3552) (70.6331, 23.8513) knots 0 0 0 1 2 2 2
  spline S91 degree 2 poles (70.6331, 23.8513) (70.811, 23.3771) (71.4705, 22.8658) (72.004, 22.8658) knots 0 0 0 1 2 2 2
  spline S92 degree 2 poles (72.004, 22.8658) (72.5079, 22.8658) (73.1674, 23.3474) (73.3526, 23.8291) knots 0 0 0 1 2 2 2
  line L150 (81.8371, 29.8164) -> (77.8802, 22.0432)
  line L151 (77.8802, 22.0432) -> (76.576, 22.0432)
  line L152 (76.576, 22.0432) -> (80.7553, 30.1128)
  line L153 (80.7553, 30.1128) -> (76.035, 30.1128)
  line L154 (76.035, 30.1128) -> (76.035, 31.1872)
  line L155 (76.035, 31.1872) -> (81.8371, 31.1872)
  line L156 (81.8371, 31.1872) -> (81.8371, 29.8164)
  line L157 (88.1357, 22.0432) -> (83.6748, 22.0432)
  line L158 (83.6748, 22.0432) -> (83.6748, 22.9769)
  line L159 (83.6748, 22.9769) -> (85.3347, 22.9769)
  line L160 (85.3347, 22.9769) -> (85.3347, 29.105)
  line L161 (85.3347, 29.105) -> (83.6748, 29.105)
  line L162 (83.6748, 29.105) -> (83.6748, 29.9424)
  spline S93 degree 2 poles (83.6748, 29.9424) (84.6159, 29.9424) (85.5051, 30.4759) (85.5644, 31.2169) knots 0 0 0 1 2 2 2
  line L163 (85.5644, 31.2169) -> (86.5129, 31.2169)
  line L164 (86.5129, 31.2169) -> (86.5129, 22.9769)
  line L165 (86.5129, 22.9769) -> (88.1357, 22.9769)
  line L166 (88.1357, 22.9769) -> (88.1357, 22.0432)
  spline S94 degree 2 poles (11.8048, 6.7952) (11.8048, 5.6244) (10.545, 4.3944) (9.4409, 4.3944) knots 0 0 0 1 2 2 2
  spline S95 degree 2 poles (9.4409, 4.3944) (9.2483, 4.3944) (8.774, 4.4314) (8.5443, 4.4685) knots 0 0 0 1 2 2 2
  line L167 (8.5443, 4.4685) -> (8.5443, 5.5059)
  line L168 (8.5443, 5.5059) -> (8.611, 5.5059)
  spline S96 degree 2 poles (8.611, 5.5059) (8.7444, 5.4762) (9.0704, 5.417) (9.2186, 5.417) knots 0 0 0 1 2 2 2
  spline S97 degree 2 poles (9.2186, 5.417) (9.6781, 5.417) (10.2783, 5.6467) (10.4191, 5.8912) knots 0 0 0 1 2 2 2
  spline S98 degree 2 poles (10.4191, 5.8912) (10.5599, 6.1135) (10.6488, 6.7878) (10.6488, 7.2695) knots 0 0 0 1 2 2 2
  line L169 (10.6488, 7.2695) -> (10.6488, 12.8937)
  line L170 (10.6488, 12.8937) -> (9.4113, 12.8937)
  line L171 (9.4113, 12.8937) -> (9.4113, 13.8496)
  line L172 (9.4113, 13.8496) -> (11.8048, 13.8496)
  line L173 (11.8048, 13.8496) -> (11.8048, 6.7952)
  line L174 (11.8122, 14.9907) -> (10.5006, 14.9907)
  line L175 (10.5006, 14.9907) -> (10.5006, 16.1912)
  line L176 (10.5006, 16.1912) -> (11.8122, 16.1912)
  line L177 (11.8122, 16.1912) -> (11.8122, 14.9907)
  spline S99 degree 2 poles (19.2296, 10.5299) (19.2296, 8.8478) (17.5994, 6.7952) (16.3693, 6.7952) knots 0 0 0 1 2 2 2
  spline S100 degree 2 poles (16.3693, 6.7952) (15.8136, 6.7952) (15.0207, 7.0694) (14.6354, 7.3065) knots 0 0 0 1 2 2 2
  line L178 (14.6354, 7.3065) -> (14.5613, 6.9879)
  line L179 (14.5613, 6.9879) -> (13.4794, 6.9879)
  line L180 (13.4794, 6.9879) -> (13.4794, 16.5394)
  line L181 (13.4794, 16.5394) -> (14.6354, 16.5394)
  line L182 (14.6354, 16.5394) -> (14.6354, 13.1308)
  spline S101 degree 2 poles (14.6354, 13.1308) (15.0726, 13.5236) (16.0878, 14.0423) (16.7324, 14.0423) knots 0 0 0 1 2 2 2
  spline S102 degree 2 poles (16.7324, 14.0423) (17.8958, 14.0423) (19.2296, 12.1823) (19.2296, 10.5299) knots 0 0 0 1 2 2 2
  spline S103 degree 2 poles (18.0366, 10.441) (18.0366, 11.671) (17.2882, 12.9456) (16.4583, 12.9456) knots 0 0 0 1 2 2 2
  spline S104 degree 2 poles (16.4583, 12.9456) (15.9914, 12.9456) (15.0281, 12.501) (14.6354, 12.1601) knots 0 0 0 1 2 2 2
  line L183 (14.6354, 12.1601) -> (14.6354, 8.2254)
  spline S105 degree 2 poles (14.6354, 8.2254) (15.0726, 8.0105) (15.7469, 7.8326) (16.147, 7.8326) knots 0 0 0 1 2 2 2
  spline S106 degree 2 poles (16.147, 7.8326) (17.0288, 7.8326) (18.0366, 9.0849) (18.0366, 10.441) knots 0 0 0 1 2 2 2
  spline S107 degree 2 poles (24.2536, 7.7141) (24.1128, 7.6103) (23.6386, 7.2398) (23.4163, 7.1287) knots 0 0 0 1 2 2 2
  spline S108 degree 2 poles (23.4163, 7.1287) (23.1125, 6.9657) (22.5419, 6.7952) (22.0232, 6.7952) knots 0 0 0 1 2 2 2
  spline S109 degree 2 poles (22.0232, 6.7952) (21.6008, 6.7952) (20.8376, 7.1139) (20.5486, 7.4029) knots 0 0 0 1 2 2 2
  spline S110 degree 2 poles (20.5486, 7.4029) (20.2744, 7.6844) (19.941, 8.5144) (19.941, 8.9738) knots 0 0 0 1 2 2 2
  spline S111 degree 2 poles (19.941, 8.9738) (19.941, 9.6852) (20.5412, 10.6929) (21.1933, 10.9819) knots 0 0 0 1 2 2 2
  spline S112 degree 2 poles (21.1933, 10.9819) (21.7713, 11.2487) (23.3422, 11.4487) (24.2536, 11.5006) knots 0 0 0 1 2 2 2
  line L184 (24.2536, 11.5006) -> (24.2536, 11.7229)
  spline S113 degree 2 poles (24.2536, 11.7229) (24.2536, 12.1231) (24.0091, 12.6195) (23.7868, 12.7603) knots 0 0 0 1 2 2 2
  spline S114 degree 2 poles (23.7868, 12.7603) (23.5645, 12.9011) (22.9272, 12.99) (22.5864, 12.99) knots 0 0 0 1 2 2 2
  spline S115 degree 2 poles (22.5864, 12.99) (22.1862, 12.99) (21.1044, 12.7529) (20.5634, 12.5232) knots 0 0 0 1 2 2 2
  line L185 (20.5634, 12.5232) -> (20.4967, 12.5232)
  line L186 (20.4967, 12.5232) -> (20.4967, 13.7014)
  spline S116 degree 2 poles (20.4967, 13.7014) (20.8154, 13.7903) (22.0084, 14.0126) (22.5938, 14.0126) knots 0 0 0 1 2 2 2
  spline S117 degree 2 poles (22.5938, 14.0126) (23.3051, 14.0126) (24.2759, 13.7903) (24.6612, 13.5013) knots 0 0 0 1 2 2 2
  spline S118 degree 2 poles (24.6612, 13.5013) (25.0391, 13.2197) (25.4096, 12.3231) (25.4096, 11.6785) knots 0 0 0 1 2 2 2
  line L187 (25.4096, 11.6785) -> (25.4096, 6.9879)
  line L188 (25.4096, 6.9879) -> (24.2536, 6.9879)
  line L189 (24.2536, 6.9879) -> (24.2536, 7.7141)
  line L190 (24.2536, 8.6774) -> (24.2536, 10.5818)
  spline S119 degree 2 poles (24.2536, 10.5818) (23.8387, 10.5447) (22.5864, 10.4187) (22.1936, 10.3002) knots 0 0 0 1 2 2 2
  spline S120 degree 2 poles (22.1936, 10.3002) (21.7342, 10.1594) (21.134, 9.574) (21.134, 9.0553) knots 0 0 0 1 2 2 2
  spline S121 degree 2 poles (21.134, 9.0553) (21.134, 8.4625) (21.8009, 7.8623) (22.4382, 7.8623) knots 0 0 0 1 2 2 2
  spline S122 degree 2 poles (22.4382, 7.8623) (22.9791, 7.8623) (23.8683, 8.3291) (24.2536, 8.6774) knots 0 0 0 1 2 2 2
  line L191 (28.2106, 6.9879) -> (27.0546, 6.9879)
  line L192 (27.0546, 6.9879) -> (27.0546, 16.5394)
  line L193 (27.0546, 16.5394) -> (28.2106, 16.5394)
  line L194 (28.2106, 16.5394) -> (28.2106, 6.9879)
  line L195 (31.0857, 6.9879) -> (29.9297, 6.9879)
  line L196 (29.9297, 6.9879) -> (29.9297, 16.5394)
  line L197 (29.9297, 16.5394) -> (31.0857, 16.5394)
  line L198 (31.0857, 16.5394) -> (31.0857, 6.9879)
  spline S123 degree 2 poles (35.7614, 6.8323) (34.1164, 6.8323) (32.3084, 8.6774) (32.3084, 10.3817) knots 0 0 0 1 2 2 2
  spline S124 degree 2 poles (32.3084, 10.3817) (32.3084, 12.0564) (34.0645, 14.0423) (35.4799, 14.0423) knots 0 0 0 1 2 2 2
  spline S125 degree 2 poles (35.4799, 14.0423) (36.1171, 14.0423) (37.1027, 13.6718) (37.4657, 13.279) knots 0 0 0 1 2 2 2
  spline S126 degree 2 poles (37.4657, 13.279) (37.8363, 12.8863) (38.229, 11.7526) (38.229, 10.93) knots 0 0 0 1 2 2 2
  line L199 (38.229, 10.93) -> (38.229, 10.3002)
  line L200 (38.229, 10.3002) -> (33.4791, 10.3002)
  spline S127 degree 2 poles (33.4791, 10.3002) (33.4791, 9.1072) (34.6796, 7.84) (35.7466, 7.84) knots 0 0 0 1 2 2 2
  spline S128 degree 2 poles (35.7466, 7.84) (36.1245, 7.84) (36.8581, 8.0105) (37.1545, 8.1439) knots 0 0 0 1 2 2 2
  spline S129 degree 2 poles (37.1545, 8.1439) (37.4657, 8.2921) (37.8955, 8.5514) (38.0363, 8.67) knots 0 0 0 1 2 2 2
  line L201 (38.0363, 8.67) -> (38.103, 8.67)
  line L202 (38.103, 8.67) -> (38.103, 7.4103)
  spline S130 degree 2 poles (38.103, 7.4103) (37.9029, 7.3288) (37.2953, 7.0916) (37.0582, 7.0249) knots 0 0 0 1 2 2 2
  spline S131 degree 2 poles (37.0582, 7.0249) (36.7247, 6.9286) (36.1764, 6.8323) (35.7614, 6.8323) knots 0 0 0 1 2 2 2
  spline S132 degree 2 poles (37.1027, 11.182) (37.0878, 11.6488) (36.8952, 12.3305) (36.7099, 12.5602) knots 0 0 0 1 2 2 2
  spline S133 degree 2 poles (36.7099, 12.5602) (36.5099, 12.8196) (35.88, 13.0938) (35.4132, 13.0938) knots 0 0 0 1 2 2 2
  spline S134 degree 2 poles (35.4132, 13.0938) (34.9537, 13.0938) (34.3091, 12.8196) (34.0423, 12.5528) knots 0 0 0 1 2 2 2
  spline S135 degree 2 poles (34.0423, 12.5528) (33.783, 12.2787) (33.5162, 11.6192) (33.4791, 11.182) knots 0 0 0 1 2 2 2
  line L203 (33.4791, 11.182) -> (37.1027, 11.182)
  line L204 (44.7869, 6.9879) -> (43.6309, 6.9879)
  line L205 (43.6309, 6.9879) -> (43.6309, 10.9004)
  spline S136 degree 2 poles (43.6309, 10.9004) (43.6309, 11.3746) (43.542, 12.1897) (43.4086, 12.4343) knots 0 0 0 1 2 2 2
  spline S137 degree 2 poles (43.4086, 12.4343) (43.2678, 12.6936) (42.7639, 12.9456) (42.3342, 12.9456) knots 0 0 0 1 2 2 2
  spline S138 degree 2 poles (42.3342, 12.9456) (41.9044, 12.9456) (40.9929, 12.4861) (40.5557, 12.1156) knots 0 0 0 1 2 2 2
  line L206 (40.5557, 12.1156) -> (40.5557, 6.9879)
  line L207 (40.5557, 6.9879) -> (39.3998, 6.9879)
  line L208 (39.3998, 6.9879) -> (39.3998, 13.8496)
  line L209 (39.3998, 13.8496) -> (40.5557, 13.8496)
  line L210 (40.5557, 13.8496) -> (40.5557, 13.0864)
  spline S139 degree 2 poles (40.5557, 13.0864) (41.0744, 13.5532) (42.0748, 14.0423) (42.638, 14.0423) knots 0 0 0 1 2 2 2
  spline S140 degree 2 poles (42.638, 14.0423) (43.6457, 14.0423) (44.7869, 12.7085) (44.7869, 11.4413) knots 0 0 0 1 2 2 2
  line L211 (44.7869, 11.4413) -> (44.7869, 6.9879)
  spline S141 degree 2 poles (56.2502, 11.0634) (56.2502, 10.2113) (55.7834, 8.6181) (55.3462, 7.9586) knots 0 0 0 1 2 2 2
  line L212 (55.3462, 7.9586) -> (52.7675, 7.9586)
  line L213 (52.7675, 7.9586) -> (52.6119, 8.67)
  spline S142 degree 2 poles (52.6119, 8.67) (52.1969, 8.3217) (51.5078, 7.9067) (50.9076, 7.9067) knots 0 0 0 1 2 2 2
  spline S143 degree 2 poles (50.9076, 7.9067) (49.9665, 7.9067) (48.7587, 9.4258) (48.7587, 10.8633) knots 0 0 0 1 2 2 2
  spline S144 degree 2 poles (48.7587, 10.8633) (48.7587, 12.3083) (50.2407, 13.9163) (51.1966, 13.9163) knots 0 0 0 1 2 2 2
  spline S145 degree 2 poles (51.1966, 13.9163) (51.6412, 13.9163) (52.2784, 13.694) (52.6045, 13.5087) knots 0 0 0 1 2 2 2
  line L214 (52.6045, 13.5087) -> (52.6045, 13.8051)
  line L215 (52.6045, 13.8051) -> (53.5752, 13.8051)
  line L216 (53.5752, 13.8051) -> (53.5752, 8.6403)
  line L217 (53.5752, 8.6403) -> (54.9683, 8.6403)
  spline S146 degree 2 poles (54.9683, 8.6403) (55.2054, 9.0775) (55.4055, 10.4632) (55.4055, 11.0264) knots 0 0 0 1 2 2 2
  spline S147 degree 2 poles (55.4055, 11.0264) (55.4055, 13.0345) (53.3603, 15.4798) (51.4411, 15.4798) knots 0 0 0 1 2 2 2
  spline S148 degree 2 poles (51.4411, 15.4798) (49.6256, 15.4798) (47.2618, 12.8344) (47.2618, 10.9449) knots 0 0 0 1 2 2 2
  spline S149 degree 2 poles (47.2618, 10.9449) (47.2618, 8.9219) (49.5589, 6.4099) (51.4115, 6.4099) knots 0 0 0 1 2 2 2
  spline S150 degree 2 poles (51.4115, 6.4099) (51.9079, 6.4099) (53.012, 6.5433) (53.5011, 6.6915) knots 0 0 0 1 2 2 2
  line L218 (53.5011, 6.6915) -> (53.5011, 5.8245)
  spline S151 degree 2 poles (53.5011, 5.8245) (52.9824, 5.6985) (51.9228, 5.6022) (51.4041, 5.6022) knots 0 0 0 1 2 2 2
  spline S152 degree 2 poles (51.4041, 5.6022) (49.2329, 5.6022) (46.38, 8.5885) (46.38, 10.9597) knots 0 0 0 1 2 2 2
  spline S153 degree 2 poles (46.38, 10.9597) (46.38, 13.2123) (49.3218, 16.3097) (51.4337, 16.3097) knots 0 0 0 1 2 2 2
  spline S154 degree 2 poles (51.4337, 16.3097) (53.6938, 16.3097) (56.2502, 13.3976) (56.2502, 11.0634) knots 0 0 0 1 2 2 2
  line L219 (52.5897, 9.4925) -> (52.5897, 12.6714)
  spline S155 degree 2 poles (52.5897, 12.6714) (52.2488, 12.8492) (51.6708, 13.0049) (51.3522, 13.0049) knots 0 0 0 1 2 2 2
  spline S156 degree 2 poles (51.3522, 13.0049) (50.6556, 13.0049) (49.8109, 11.9674) (49.8109, 10.8782) knots 0 0 0 1 2 2 2
  spline S157 degree 2 poles (49.8109, 10.8782) (49.8109, 9.9) (50.4482, 8.8552) (51.1521, 8.8552) knots 0 0 0 1 2 2 2
  spline S158 degree 2 poles (51.1521, 8.8552) (51.5226, 8.8552) (52.2562, 9.2109) (52.5897, 9.4925) knots 0 0 0 1 2 2 2
  line L220 (63.1786, 6.9879) -> (62.0227, 6.9879)
  line L221 (62.0227, 6.9879) -> (62.0227, 7.7437)
  spline S159 degree 2 poles (62.0227, 7.7437) (61.4891, 7.2769) (60.5332, 6.7952) (59.9404, 6.7952) knots 0 0 0 1 2 2 2
  spline S160 degree 2 poles (59.9404, 6.7952) (59.4958, 6.7952) (58.7029, 7.0916) (58.414, 7.4103) knots 0 0 0 1 2 2 2
  spline S161 degree 2 poles (58.414, 7.4103) (58.1176, 7.7289) (57.7915, 8.6996) (57.7915, 9.3962) knots 0 0 0 1 2 2 2
  line L222 (57.7915, 9.3962) -> (57.7915, 13.8496)
  line L223 (57.7915, 13.8496) -> (58.9475, 13.8496)
  line L224 (58.9475, 13.8496) -> (58.9475, 9.9371)
  spline S162 degree 2 poles (58.9475, 9.9371) (58.9475, 9.3887) (59.029, 8.67) (59.1698, 8.4032) knots 0 0 0 1 2 2 2
  spline S163 degree 2 poles (59.1698, 8.4032) (59.3106, 8.1365) (59.7922, 7.8919) (60.2442, 7.8919) knots 0 0 0 1 2 2 2
  spline S164 degree 2 poles (60.2442, 7.8919) (60.6666, 7.8919) (61.6225, 8.3736) (62.0227, 8.7218) knots 0 0 0 1 2 2 2
  line L225 (62.0227, 8.7218) -> (62.0227, 13.8496)
  line L226 (62.0227, 13.8496) -> (63.1786, 13.8496)
  line L227 (63.1786, 13.8496) -> (63.1786, 6.9879)
  spline S165 degree 2 poles (67.5802, 6.8323) (66.8688, 6.8323) (65.6906, 7.2695) (65.2683, 7.7141) knots 0 0 0 1 2 2 2
  spline S166 degree 2 poles (65.2683, 7.7141) (64.8459, 8.1513) (64.379, 9.4999) (64.379, 10.4039) knots 0 0 0 1 2 2 2
  spline S167 degree 2 poles (64.379, 10.4039) (64.379, 11.308) (64.8607, 12.6269) (65.2683, 13.0715) knots 0 0 0 1 2 2 2
  spline S168 degree 2 poles (65.2683, 13.0715) (65.6758, 13.5236) (66.8836, 14.0052) (67.5802, 14.0052) knots 0 0 0 1 2 2 2
  spline S169 degree 2 poles (67.5802, 14.0052) (68.1434, 14.0052) (69.1956, 13.6866) (69.6031, 13.4791) knots 0 0 0 1 2 2 2
  line L228 (69.6031, 13.4791) -> (69.6031, 12.1823)
  line L229 (69.6031, 12.1823) -> (69.5364, 12.1823)
  spline S170 degree 2 poles (69.5364, 12.1823) (69.4105, 12.2861) (69.0251, 12.5528) (68.751, 12.6936) knots 0 0 0 1 2 2 2
  spline S171 degree 2 poles (68.751, 12.6936) (68.5064, 12.8122) (67.8544, 12.9974) (67.558, 12.9974) knots 0 0 0 1 2 2 2
  spline S172 degree 2 poles (67.558, 12.9974) (66.6613, 12.9974) (65.5721, 11.6414) (65.5721, 10.4039) knots 0 0 0 1 2 2 2
  spline S173 degree 2 poles (65.5721, 10.4039) (65.5721, 9.1961) (66.6243, 7.84) (67.558, 7.84) knots 0 0 0 1 2 2 2
  spline S174 degree 2 poles (67.558, 7.84) (68.1211, 7.84) (69.1437, 8.3069) (69.5364, 8.67) knots 0 0 0 1 2 2 2
  line L230 (69.5364, 8.67) -> (69.6031, 8.67)
  line L231 (69.6031, 8.67) -> (69.6031, 7.3732)
  spline S175 degree 2 poles (69.6031, 7.3732) (69.4327, 7.2917) (68.914, 7.062) (68.7065, 7.0101) knots 0 0 0 1 2 2 2
  spline S176 degree 2 poles (68.7065, 7.0101) (68.4101, 6.9212) (67.9433, 6.8323) (67.5802, 6.8323) knots 0 0 0 1 2 2 2
  spline S177 degree 2 poles (72.5079, 6.8249) (71.8187, 6.8249) (70.6257, 7.1954) (70.233, 7.4029) knots 0 0 0 1 2 2 2
  line L232 (70.233, 7.4029) -> (70.233, 8.6996)
  line L233 (70.233, 8.6996) -> (70.2923, 8.6996)
  spline S178 degree 2 poles (70.2923, 8.6996) (70.4405, 8.5811) (70.8406, 8.2995) (71.1741, 8.1439) knots 0 0 0 1 2 2 2
  spline S179 degree 2 poles (71.1741, 8.1439) (71.4631, 8.0031) (72.1744, 7.7956) (72.5523, 7.7956) knots 0 0 0 1 2 2 2
  spline S180 degree 2 poles (72.5523, 7.7956) (72.8265, 7.7956) (73.4564, 7.9216) (73.6046, 8.0253) knots 0 0 0 1 2 2 2
  spline S181 degree 2 poles (73.6046, 8.0253) (73.8194, 8.1661) (74.0121, 8.4847) (74.0121, 8.8108) knots 0 0 0 1 2 2 2
  spline S182 degree 2 poles (74.0121, 8.8108) (74.0121, 9.2183) (73.5675, 9.6407) (72.9969, 9.7815) knots 0 0 0 1 2 2 2
  spline S183 degree 2 poles (72.9969, 9.7815) (72.7746, 9.8334) (72.0633, 9.9816) (71.7595, 10.0631) knots 0 0 0 1 2 2 2
  spline S184 degree 2 poles (71.7595, 10.0631) (70.974, 10.2928) (70.2626, 11.2413) (70.2626, 11.9156) knots 0 0 0 1 2 2 2
  spline S185 degree 2 poles (70.2626, 11.9156) (70.2626, 12.8492) (71.6631, 14.0126) (72.8191, 14.0126) knots 0 0 0 1 2 2 2
  spline S186 degree 2 poles (72.8191, 14.0126) (73.3897, 14.0126) (74.5456, 13.731) (74.9384, 13.5161) knots 0 0 0 1 2 2 2
  line L234 (74.9384, 13.5161) -> (74.9384, 12.2787)
  line L235 (74.9384, 12.2787) -> (74.8791, 12.2787)
  spline S187 degree 2 poles (74.8791, 12.2787) (74.4345, 12.6343) (73.3526, 13.0419) (72.7969, 13.0419) knots 0 0 0 1 2 2 2
  spline S188 degree 2 poles (72.7969, 13.0419) (72.2263, 13.0419) (71.4408, 12.5602) (71.4408, 12.0786) knots 0 0 0 1 2 2 2
  spline S189 degree 2 poles (71.4408, 12.0786) (71.4408, 11.6414) (71.9077, 11.219) (72.4264, 11.0856) knots 0 0 0 1 2 2 2
  spline S190 degree 2 poles (72.4264, 11.0856) (72.6783, 11.019) (73.3156, 10.8856) (73.6638, 10.8041) knots 0 0 0 1 2 2 2
  spline S191 degree 2 poles (73.6638, 10.8041) (74.4197, 10.6114) (75.1903, 9.7296) (75.1903, 8.9664) knots 0 0 0 1 2 2 2
  spline S192 degree 2 poles (75.1903, 8.9664) (75.1903, 8.5218) (74.842, 7.7363) (74.5012, 7.4473) knots 0 0 0 1 2 2 2
  spline S193 degree 2 poles (74.5012, 7.4473) (74.1381, 7.1435) (73.2118, 6.8249) (72.5079, 6.8249) knots 0 0 0 1 2 2 2
  line L236 (81.5407, 6.9879) -> (80.3848, 6.9879)
  line L237 (80.3848, 6.9879) -> (80.3848, 7.6844)
  spline S194 degree 2 poles (80.3848, 7.6844) (80.118, 7.4621) (79.7253, 7.1657) (79.4585, 7.0398) knots 0 0 0 1 2 2 2
  spline S195 degree 2 poles (79.4585, 7.0398) (79.214, 6.9212) (78.6878, 6.7952) (78.3396, 6.7952) knots 0 0 0 1 2 2 2
  spline S196 degree 2 poles (78.3396, 6.7952) (77.7764, 6.7952) (76.8279, 7.2621) (76.4945, 7.7141) knots 0 0 0 1 2 2 2
  spline S197 degree 2 poles (76.4945, 7.7141) (76.161, 8.1661) (75.7905, 9.4999) (75.7905, 10.3669) knots 0 0 0 1 2 2 2
  spline S198 degree 2 poles (75.7905, 10.3669) (75.7905, 11.2709) (76.2574, 12.5899) (76.6649, 13.0864) knots 0 0 0 1 2 2 2
  spline S199 degree 2 poles (76.6649, 13.0864) (77.0428, 13.531) (78.1025, 14.0423) (78.6878, 14.0423) knots 0 0 0 1 2 2 2
  spline S200 degree 2 poles (78.6878, 14.0423) (79.1991, 14.0423) (79.9624, 13.8125) (80.3848, 13.5754) knots 0 0 0 1 2 2 2
  line L238 (80.3848, 13.5754) -> (80.3848, 16.5394)
  line L239 (80.3848, 16.5394) -> (81.5407, 16.5394)
  line L240 (81.5407, 16.5394) -> (81.5407, 6.9879)
  line L241 (80.3848, 8.6552) -> (80.3848, 12.6195)
  spline S201 degree 2 poles (80.3848, 12.6195) (79.955, 12.827) (79.2732, 12.9826) (78.8805, 12.9826) knots 0 0 0 1 2 2 2
  spline S202 degree 2 poles (78.8805, 12.9826) (77.9913, 12.9826) (76.9835, 11.6488) (76.9835, 10.3891) knots 0 0 0 1 2 2 2
  spline S203 degree 2 poles (76.9835, 10.3891) (76.9835, 9.1739) (77.7542, 7.8919) (78.6063, 7.8919) knots 0 0 0 1 2 2 2
  spline S204 degree 2 poles (78.6063, 7.8919) (79.0584, 7.8919) (79.9772, 8.3069) (80.3848, 8.6552) knots 0 0 0 1 2 2 2
  line L242 (85.0086, 6.9879) -> (83.5414, 6.9879)
  line L243 (83.5414, 6.9879) -> (83.5414, 8.7367)
  line L244 (83.5414, 8.7367) -> (85.0086, 8.7367)
  line L245 (85.0086, 8.7367) -> (85.0086, 6.9879)
  spline S205 degree 2 poles (90.003, 6.8323) (88.358, 6.8323) (86.5499, 8.6774) (86.5499, 10.3817) knots 0 0 0 1 2 2 2